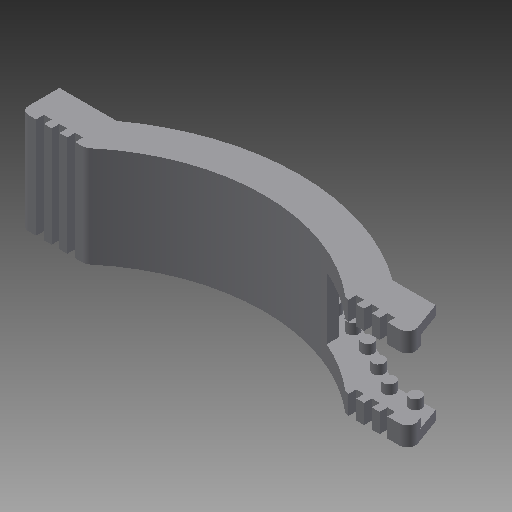
# Autodesk Inventor part: VEX Claw Gripper
Saved by Autodesk Inventor 2018 (Build 220112000, 112)
## iProperties
Created: 2011-04-06
Part Number: VEX Claw Gripper
Document SubType Name: Modeling
Designer: Phillip
Density: 1 g/cm^3
Mass: 2.73206 g
Surface Area: 37.4849 cm^2
Volume: 2.73206 cm^3
Material: Generic
Appearance: Default
Author: Phillip
Autodesk Inventor part; units mm, degrees
ref_plane "Work Plane2" through (0, 0, 0) normal (0, 0, 1) x (1, 0, 0)
sketch "Sketch3" plane through (0, 0, 0) normal (0, 0, 1) x (1, 0, 0)
  arc A0 (18.4699, -20.8931) -> (63.3521, -20.8931) centre (40.911, 9.7976) ccw projected
  line L0 (18.4699, -20.8931) -> (11.4586, -20.8931) projected
  line L1 (11.4586, -20.8931) -> (10.0439, -17.0323) projected
  line L2 (10.0439, -17.0323) -> (19.7685, -17.0323) projected
  arc A1 (19.7685, -17.0323) -> (62.0536, -17.0323) centre (40.911, 9.7976) ccw projected
  line L3 (62.0536, -17.0323) -> (72.661, -17.0323) projected
  line L4 (72.661, -17.0323) -> (72.661, -20.8931) projected
  line L5 (72.661, -20.8931) -> (63.3521, -20.8931) projected
  point P0 (0, 0)
ref_plane "Work Plane3" through (-19.825, 4.9027, -1.6002) normal (0, 0, 1) x (1, 0, 0)
extrude "Extrusion1" add sketch "Sketch3" against normal up to surface (1.6002 mm away)
sketch "Sketch4" plane through (40.911, 9.7976, -1.6002) normal (0, 0, -1) x (-1, 0, 0)
  circle A0 centre (-29.2608, -29.7001) radius 0.9906 projected
  circle A1 centre (-25.004, -29.7001) radius 0.9906 projected
  circle A2 centre (-21.0031, -30.4967) radius 0.9906 projected
  circle A3 centre (-17.3663, -32.7046) radius 0.9906 projected
  circle A4 centre (-13.5003, -34.4807) radius 0.9906 projected
  circle A5 centre (-9.456, -35.8017) radius 0.9906 projected
  circle A6 centre (-5.287, -36.65) radius 0.9906 projected
  circle A7 centre (-1.0481, -37.0146) radius 0.9906 projected
  circle A8 centre (-1.0481, -37.0146) radius 0.9906 projected
  circle A9 centre (3.2046, -36.8905) radius 0.9906 projected
  circle A10 centre (7.415, -36.2794) radius 0.9906 projected
  circle A11 centre (11.5275, -35.1894) radius 0.9906 projected
  circle A12 centre (15.4878, -33.6349) radius 0.9906 projected
  circle A13 centre (19.2437, -31.6363) radius 0.9906 projected
  circle A14 centre (22.9075, -29.7001) radius 0.9906 projected
  circle A15 centre (27.1643, -29.7001) radius 0.9906 projected
  point P0 (40.911, -9.7975)
ref_plane "Work Plane4" through (-39.3728, -16.3857, -3.302) normal (0, 0, -1) x (0, 1, 0)
extrude "Extrusion2" add sketch "Sketch4" along normal up to surface (1.7018 mm away)
ref_plane "Work Plane5" through (41.0844, 8.0897, -8.1915) normal (0, 0, -1) x (-1, 0, 0)
mirror "Mirror1" about plane through (41.0844, 8.0897, -8.1915) normal (0, 0, -1) of "Extrusion1", "Extrusion2"
sketch "Sketch6" plane through (0, 0, 0) normal (0, 0, 1) x (1, 0, 0)
  line L0 (63.3521, -20.8931) -> (72.661, -20.8931) projected
  line L1 (72.661, -17.0323) -> (62.0536, -17.0323) projected
  arc A0 (19.7685, -17.0323) -> (62.0536, -17.0323) centre (40.911, 9.7976) ccw projected
  line L2 (19.7685, -17.0323) -> (10.0439, -17.0323) projected
  line L3 (10.0439, -17.0323) -> (11.4586, -20.8931) projected
  line L4 (11.4586, -20.8931) -> (18.4699, -20.8931) projected
  line L5 (72.661, -17.0323) -> (72.661, -14.5431)
  line L6 (72.661, -14.5431) -> (62.0536, -14.5431)
  line L7 (10.0439, -17.0323) -> (9.1317, -14.5431)
  line L8 (19.7685, -14.5431) -> (9.1317, -14.5431)
  arc A1 (19.7685, -14.5431) -> (62.0536, -14.5431) centre (40.911, 9.7976) ccw
  point P0 (0, 0)
  dimension "d8" = 6.35
  constraints: 8 end point, 2 perpendicular, 2 point on circle, 2 vertical alignment, 1 centre point, 1 collinear, 1 concentric, 1 parallel
  measures "d8" distance between parallel lines of L6 L0
extrude "Extrusion3" add sketch "Sketch6" against normal up to surface (16.383 mm away)
sketch "Sketch7" plane through (9.1317, -14.5431, 0) normal (0, 1, 0) x (1, 0, 0)
  line L0 (0, 0) -> (0, 16.383) projected
  line L1 (10.6367, 0) -> (10.6367, 16.383) projected
  line L2 (10.6367, 3.1115) -> (0.9122, 3.1115) projected
  line L3 (18.9409, 3.1115) -> (10.6367, 3.1115) projected
  line L4 (18.9409, 13.2715) -> (18.9409, 3.1115) projected
  line L5 (10.6367, 13.2715) -> (18.9409, 13.2715) projected
  line L6 (0.9122, 13.2715) -> (10.6367, 13.2715) projected
  line L7 (0.9122, 3.1115) -> (0, 3.1115)
  line L8 (0.9122, 13.2715) -> (0, 13.2715)
  point P0 (-9.1317, 0)
  constraints: 4 end point, 2 perpendicular, 2 point on line
ref_plane "Work Plane6" through (-30.3687, -13.9561, -13.462) normal (-0.2426, 0.9701, 0) x (0, 0, 1)
ref_plane "Work Plane7" through (-0.4999, -47.0812, -13.462) normal (-0.2426, 0.9701, 0) x (0, 0, 1)
extrude "Extrusion7" cut sketch "Sketch7" against normal up to surface surface through (-0.4999, -47.0812, -13.462) normal (-0.2426, 0.9701, 0)
fillet "Fillet1" radius 1.27 6 edges at (72.661, -14.5431, -8.1915) (62.0536, -14.5431, -8.1915) (19.7685, -14.5431, -14.8273) (19.7685, -14.5431, -1.5558) (9.1317, -14.5431, -1.5558) (9.1317, -14.5431, -14.8273)
sketch "Sketch8" plane through (0, 0, 0) normal (0, 0, 1) x (1, 0, 0)
  line L0 (71.391, -14.5431) -> (62.5229, -14.5431) projected
  line L1 (70.121, -14.5431) -> (68.851, -14.5431)
  line L2 (68.851, -14.5431) -> (68.851, -15.8131)
  line L3 (68.851, -15.8131) -> (70.121, -15.8131)
  line L4 (70.121, -15.8131) -> (70.121, -14.5431)
  point P0 (72.661, -15.8131)
  point P1 (0, 0)
  dimension "d14" = 1.27
  dimension "d15" = 2.54
  dimension "d16" = 1.27
  constraints: 8 end point, 2 parallel, 1 horizontal, 1 perpendicular, 1 point on line
  measures "d14" distance of L1.start L1.end
  measures "d15" distance of point (72.661, -15.813) L3.end
  measures "d16" distance of L1.end L2.end
extrude "Extrusion5" cut sketch "Sketch8" against normal up to next
pattern_linear "Rectangular Pattern1" count 3 spacing 2.54 along (-1, 0, 0) of "Extrusion5"
sketch "Sketch9" plane through (0, 0, 0) normal (0, 0, 1) x (1, 0, 0)
  line L0 (19.2991, -14.5431) -> (18.0291, -14.5431)
  line L1 (18.0291, -14.5431) -> (18.0291, -15.8131)
  line L2 (18.0291, -15.8131) -> (19.2991, -15.8131)
  line L3 (19.2991, -15.8131) -> (19.2991, -14.5431)
  point P0 (3.3198, 0.6098)
  point P1 (0, 0)
  dimension "d22" = 1.27
  dimension "d28" = 1.27
  constraints: 6 end point, 3 parallel, 1 horizontal, 1 perpendicular
  measures "d22" distance of L2.end L1.end
  measures "d28" distance of L0.end L1.end
extrude "Extrusion6" cut sketch "Sketch9" against normal up to surface (16.383 mm away)
pattern_linear "Rectangular Pattern2" count 3 spacing 2.54 along (-1, 0, 0) of "Extrusion6"
equation "\"d28\" = d22"
body "Solid1"
